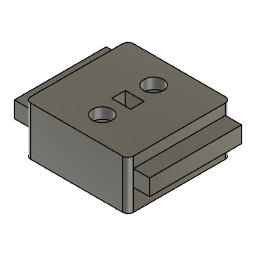
Korry Horizontal (Autodesk Fusion 360 design; units mm, degrees)
Autodesk Fusion 360 part; units mm, degrees
sketch "Sketch1" plane through (0, 0, 0) normal (0, 0, 1) x (1, 0, 0)
  line L0 (1, 0) -> (18, 0)
  line L1 (19, 1) -> (19, 18)
  line L2 (18, 19) -> (1, 19)
  line L3 (0, 18) -> (0, 1)
  arc A0 (1, 19) -> (0, 18) centre (1, 18) ccw
  arc A1 (19, 18) -> (18, 19) centre (18, 18) ccw
  arc A2 (18, 0) -> (19, 1) centre (18, 1) ccw
  arc A3 (0, 1) -> (1, 0) centre (1, 1) ccw
  line L4 (18.7071, 18.7071) -> (0.2929, 0.2929) construction
  line L5 (18.7071, 0.2929) -> (0.2929, 18.7071) construction
  line L6 (2, 17) -> (17, 17)
  line L7 (17, 17) -> (17, 2)
  line L8 (17, 2) -> (2, 2)
  line L9 (2, 2) -> (2, 17)
  line L10 (17, 17) -> (2, 2) construction
  line L11 (2, 17) -> (17, 2) construction
  point P0 (19, 0)
  point P1 (0, 19)
  point P2 (9.5, 9.5)
  point P3 (9.5, 9.5)
  dimension "d1" = 19
  dimension "d2" = 19
  dimension "d3" = 1
  dimension "d4" = 1
  dimension "d5" = 1
  dimension "d6" = 1
  dimension "d7" = 15
  dimension "d8" = 15
  constraint horizontal L0
  constraint vertical L1
  constraint horizontal L2
  constraint vertical L3
  constraint coincident P1 L2
  constraint coincident P1 L3
  constraint tangent L2 A0
  constraint tangent L3 A0
  constraint tangent L1 A1
  constraint tangent L2 A1
  constraint coincident P0 L0
  constraint coincident P0 L1
  constraint tangent L0 A2
  constraint tangent L1 A2
  constraint coincident origin L0
  constraint coincident origin L3
  constraint tangent L0 A3
  constraint tangent L3 A3
  constraint midpoint A1 L4.start
  constraint midpoint A3 L4.end
  constraint midpoint A2 L5.start
  constraint midpoint A0 L5.end
  constraint midpoint L5 P3
  constraint horizontal L6
  constraint vertical L7
  constraint horizontal L8
  constraint vertical L9
  constraint midpoint L11 P3
  measures "d1" distance of origin P0
  measures "d2" distance of origin P1
  measures "d3" radius of A0
  measures "d4" radius of A1
  measures "d5" radius of A2
  measures "d6" radius of A3
  measures "d7" distance of L6.start L6.end
  measures "d8" distance of L6.start L8.end
extrude "Extrude1" add sketch "Sketch1" along normal blind 3 makes body 1
sketch "Sketch2" plane through (0, 0, 3) normal (0, 0, 1) x (-1, 0, 0)
  line L0 (-17, -2) -> (-2, -2)
  line L1 (-2, -2) -> (-2, -17)
  line L2 (-2, -17) -> (-17, -17)
  line L3 (-17, -17) -> (-17, -2)
  arc A0 (0, -1) -> (-1, 0) centre (-1, -1) ccw
  line L4 (-1, 0) -> (-18, 0)
  arc A1 (-18, 0) -> (-19, -1) centre (-18, -1) ccw
  line L5 (-19, -1) -> (-19, -18)
  arc A2 (-19, -18) -> (-18, -19) centre (-18, -18) ccw
  line L6 (-18, -19) -> (-1, -19)
  arc A3 (-1, -19) -> (0, -18) centre (-1, -18) ccw
  line L7 (0, -18) -> (0, -1)
  line L8 (-17, -2) -> (-2, -17) construction
  line L9 (-2, -2) -> (-17, -17) construction
  line L10 (-9.5, -9.5) -> (-17, -9.5) construction
  line L11 (-9.5, -9.5) -> (-2, -9.5) construction
  line L12 (-17, -11.5) -> (-2, -11.5)
  line L13 (-17, -7.5) -> (-2, -7.5)
  line L14 (-2, -7.5) -> (-2, -11.5)
  line L15 (-17, -11.5) -> (-17, -7.5)
  line L16 (-7.75, -10.75) -> (-11.25, -10.75)
  line L17 (-11.25, -10.75) -> (-11.25, -8.25)
  line L18 (-11.25, -8.25) -> (-7.75, -8.25)
  line L19 (-7.75, -8.25) -> (-7.75, -10.75)
  line L20 (-11.25, -8.25) -> (-7.75, -10.75) construction
  line L21 (-11.25, -10.75) -> (-7.75, -8.25) construction
  point P0 (-9.5, -9.5)
  point P1 (-9.5, -9.5)
  dimension "d11" = 2
  dimension "d12" = 2
  dimension "d13" = 3.5
  dimension "d14" = 2.5
  constraint coincident L0.start L3.end
  constraint coincident L1.end L2.start
  constraint coincident L0.end L1.start
  constraint coincident L2.end L3.start
  constraint midpoint L9 P1
  constraint midpoint L3 L10.end
  constraint midpoint L1 L11.end
  constraint coincident L1 L12.end
  constraint perpendicular L1 L12
  constraint coincident L1 L13.end
  constraint perpendicular L1 L13
  constraint perpendicular L13 L15
  constraint horizontal L16
  constraint vertical L17
  constraint horizontal L18
  constraint vertical L19
  constraint midpoint L20 P1
  constraint coincident P1 P0
  measures "d11" distance of L10.end L12.start
  measures "d12" distance of L10.end L13.start
  measures "d13" distance of L16.start L16.end
  measures "d14" distance of L16.start L18.end
extrude "Extrude2" add sketch "Sketch2" along normal blind 4 separate body contours L1 L3 L12 L13 L14 L15 makes body 2
extrude "Extrude3" add 1 faces at (0.6667, 7, 3) along direction (0, 0, 1) blind 4 on bodies 1 bodies 1 2
sketch "Sketch3" plane through (0, 11.5, 0) normal (0, 1, 0) x (-1, 0, 0)
  line L0 (-17, 3) -> (-2, 3)
  line L1 (-2, 3) -> (-2, 7)
  line L2 (-2, 7) -> (-17, 7)
  line L3 (-17, 7) -> (-17, 3)
sketch "Sketch4" plane through (0, 0, 7) normal (0, 0, 1) x (-1, 0, 0)
  line L0 (-17, -7.5) -> (-17, -2)
  line L1 (-17, -2) -> (-2, -2)
  line L2 (-2, -2) -> (-2, -7.5)
  line L3 (-2, -7.5) -> (-17, -7.5)
  line L4 (-11.25, -8.25) -> (-7.75, -8.25)
  line L5 (-7.75, -8.25) -> (-7.75, -10.75)
  line L6 (-7.75, -10.75) -> (-11.25, -10.75)
  line L7 (-11.25, -10.75) -> (-11.25, -8.25)
  line L8 (-17, -11.5) -> (-2, -11.5)
  line L9 (-2, -11.5) -> (-2, -17)
  line L10 (-2, -17) -> (-17, -17)
  line L11 (-17, -17) -> (-17, -11.5)
  arc A0 (0, -1) -> (-1, 0) centre (-1, -1) ccw
  line L12 (-1, 0) -> (-18, 0)
  arc A1 (-18, 0) -> (-19, -1) centre (-18, -1) ccw
  line L13 (-19, -1) -> (-19, -18)
  arc A2 (-19, -18) -> (-18, -19) centre (-18, -18) ccw
  line L14 (-18, -19) -> (-1, -19)
  arc A3 (-1, -19) -> (0, -18) centre (-1, -18) ccw
  line L15 (0, -18) -> (0, -1)
  line L16 (-17, -11.5) -> (-2, -17) construction
  line L17 (-2, -11.5) -> (-17, -17) construction
  line L18 (-17, -2) -> (-2, -7.5) construction
  line L19 (-2, -2) -> (-17, -7.5) construction
  line L20 (-17, -11.5) -> (-2, -11.5)
  line L21 (-2, -11.5) -> (-17, -17) construction
  line L22 (-2, -17) -> (-17, -17)
  circle A4 centre (-9.5, -14.25) radius 1.8
  line L23 (-2, -11.5) -> (-2, -17)
  line L24 (-17, -11.5) -> (-2, -17) construction
  line L25 (-17, -17) -> (-17, -11.5)
  line L26 (-2, -7.5) -> (-17, -7.5)
  circle A5 centre (-9.5, -4.75) radius 1.8
  line L27 (-2, -2) -> (-2, -7.5)
  line L28 (-2, -2) -> (-17, -7.5) construction
  line L29 (-17, -7.5) -> (-17, -2)
  line L30 (-17, -2) -> (-2, -2)
  line L31 (-17, -2) -> (-2, -7.5) construction
  point P0 (-9.5, -14.25)
  point P1 (-9.5, -4.75)
  point P2 (-9.5, -14.25)
  point P3 (-9.5, -4.75)
  dimension "d22" = 15
  dimension "d23" = 5.5
  dimension "d24" = 3.6
  dimension "d25" = 15
  dimension "d26" = 5.5
  dimension "d27" = 3.6
  constraint coincident L8.start L11.end
  constraint coincident L9.end L10.start
  constraint coincident L8.end L9.start
  constraint coincident L10.end L11.start
  constraint coincident L0.end L1.start
  constraint coincident L2.end L3.start
  constraint coincident L1.end L2.start
  constraint coincident L0.start L3.end
  constraint midpoint L17 P2
  constraint midpoint L19 P3
  constraint horizontal L22
  constraint vertical L25
  constraint horizontal L20
  constraint vertical L23
  constraint midpoint P2 L24
  constraint coincident P2 P0
  constraint horizontal L26
  constraint vertical L29
  constraint horizontal L30
  constraint vertical L27
  constraint midpoint P3 L31
  constraint coincident P3 P1
  measures "d22" distance of L10.end L9.end
  measures "d23" distance of L9.end L8.end
  measures "d24" diameter of A4
  measures "d25" distance of L0.start L2.end
  measures "d26" distance of L2.end L1.end
  measures "d27" diameter of A5
extrude "Extrude4" add sketch "Sketch4" along normal blind 2 separate body contours L0 L1 L2 L3 L26 L27 L29 L30 | L8 L9 L10 L11 L20 L22 L23 L25 makes body 3 at (3.9, 14.25, 7) makes body 4 at (15.1, 4.75, 7)
extrude "Extrude5" add 1 faces at (15.0833, 9.9167, 7) along direction (0, 0, 1) blind 2 on bodies 1 bodies 1 3 4
sketch "Sketch5" plane through (19, 0, 0) normal (1, 0, 0) x (0, 1, 0)
  line L0 (1, 0) -> (18, 0)
  line L1 (18, 0) -> (18, 9)
  line L2 (18, 9) -> (1, 9)
  line L3 (1, 9) -> (1, 0)
  line L4 (18, 0) -> (18, 4) construction
  line L5 (18, 4) -> (1, 4)
  line L6 (1, 4) -> (1, 7)
  line L7 (1, 7) -> (18, 7)
  line L8 (18, 7) -> (18, 4)
  dimension "d32" = 4
  dimension "d33" = 3
  constraint coincident L0.end L1.start
  constraint perpendicular L0 L4
  constraint coincident L3 L5.end
  constraint perpendicular L3 L5
  constraint perpendicular L5 L6
  constraint coincident L1 L7.end
  constraint perpendicular L1 L7
  measures "d32" distance of L0.end L4.end
  measures "d33" distance of L5.end L6.end
extrude "Extrude6" add sketch "Sketch5" along normal blind 3 contours L1 L3 L5 L6 L7 L8 bodies 1
sketch "Sketch6" plane through (0, 0, 0) normal (-1, 0, 0) x (0, -1, 0)
  line L0 (-18, 0) -> (-1, 0)
  line L1 (-1, 0) -> (-1, 9)
  line L2 (-1, 9) -> (-18, 9)
  line L3 (-18, 9) -> (-18, 0)
  line L4 (-1, 0) -> (-1, 4) construction
  line L5 (-1, 4) -> (-18, 4)
  line L6 (-18, 4) -> (-18, 7)
  line L7 (-18, 7) -> (-1, 7)
  line L8 (-1, 7) -> (-1, 4)
  dimension "d36" = 4
  dimension "d37" = 3
  constraint coincident L0.end L1.start
  constraint perpendicular L0 L4
  constraint coincident L3 L5.end
  constraint perpendicular L3 L5
  constraint perpendicular L5 L6
  constraint coincident L1 L7.end
  constraint perpendicular L1 L7
  measures "d36" distance of L0.end L4.end
  measures "d37" distance of L5.end L6.end
extrude "Extrude7" add sketch "Sketch6" along normal blind 3 contours L1 L3 L5 L6 L7 L8 bodies 1
